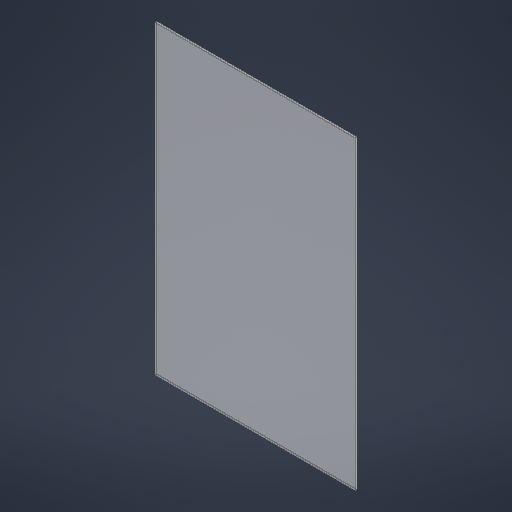
# Autodesk Inventor part: PLANCHA DE CRISTAL TRANSPARENTE 3300x2140 mm
Saved by Autodesk Inventor 2025 (Build 290162000, 162)
## iProperties
Created: 2026-02-16
Part Number: PLANCHA DE CRISTAL TRANSPARENTE 3300x2140 mm
Material: Cristal
Document SubType Name: Modeling
Designer: Frank
Density: 2.18 g/cm^3
Appearance: Transparente - Claro
Author: Frank
Autodesk Inventor part; units mm, degrees
ref_plane "YZ Plane" through (0, 0, 0) normal (1, 0, 0) x (0, 1, 0)
ref_plane "XZ Plane" through (0, 0, 0) normal (0, 1, 0) x (-1, 0, 0)
ref_plane "XY Plane" through (0, 0, 0) normal (0, 0, 1) x (1, 0, 0)
sketch "Boceto1" plane through (0, 0, 0) normal (0, 0, 1) x (1, 0, 0)
  line L0 (-625, 953) -> (0, 953)
  line L1 (0, 953) -> (0, 0)
  line L2 (0, 0) -> (-625, 0)
  line L3 (-625, 0) -> (-625, 953)
  dimension "d2" = 625
  dimension "d3" = 953
  constraints: 8 end point, 2 parallel, 2 point on line, 1 horizontal, 1 perpendicular
  measures "d2" distance of L0.start L0.end
  measures "d3" distance of L2.end L0.start
extrude "Extrusión1" add sketch "Boceto1" along normal blind 6
